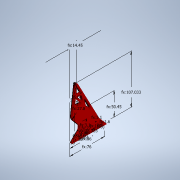
# Autodesk Inventor part: WeaponMountBasePlateV1
Saved by Autodesk Inventor 2020 (Build 240168000, 168)
## iProperties
Created: 2024-02-06
Part Number: WeaponMountBasePlateV1
Material: PETG
Document SubType Name: Modeling
Designer: smz3rm
Density: 1 g/cm^3
Appearance: Generic
Mass: 9.49681 g
Surface Area: 76.5782 cm^2
Volume: 9.49681 cm^3
WeaponHeight: 50.450 mm
SlotWidth: 6.000 mm
WeaponBite: 30.000 mm
WeaponMotorDia: 27.800 mm
SlotSpacing: 16.333 mm
SlotOffset: 2.000 mm
SlotHeight: 4.000 mm
SlotTolerance: 0.800 mm
WeaponMountBaseThinThickness: 1.000 mm
Height: 30.000 mm
BaseThickness: 3.000 mm
SideThickness: 6.000 mm
TopThickness: 1.000 mm
M3ScrewInsertBrim: 8.000 mm
M3ScrewDia: 3.100 mm
M3ScrewInsertDia: 4.000 mm
VM3ScrewInsertDia: 3.750 mm
FrontAngle: 45.00 deg
WeaponOpeningWidth: 15.000 mm
WeaponAssemblyWidth: 35.000 mm
WeaponCenterToMotorBack: 32.000 mm
WeaponMountThickness: 5.000 mm
WeaponDia: 88.900 mm
WeaponThickness: 3.000 mm
WeaponClearance: 10.000 mm
WeaponMotorShaftDia: 4.500 mm
WeaponMountWidth: 55.000 mm
Author: smz3rm
Autodesk Inventor part; units mm, degrees
ref_plane "YZ Plane" through (0, 0, 0) normal (1, 0, 0) x (0, 1, 0)
ref_plane "XZ Plane" through (0, 0, 0) normal (0, 1, 0) x (-1, 0, 0)
ref_plane "XY Plane" through (0, 0, 0) normal (0, 0, 1) x (1, 0, 0)
sketch "Sketch1" plane through (0, 0, 0) normal (1, 0, 0) x (0, 1, 0)
  line L0 (0, 0) -> (27, -27)
  line L1 (27, -27) -> (0, -27)
  line L2 (0, -27) -> (0, 0)
  line L3 (0, -76) -> (0, -27)
  arc A0 (52.1657, -0.6563) -> (59.496, -25.0037) centre (50.45, -14.45) ccw
  line L4 (6.4, -27) -> (1.6, -27)
  line L5 (1.6, -27) -> (1.6, -33.8)
  line L6 (1.6, -33.8) -> (6.4, -33.8)
  line L7 (6.4, -33.8) -> (6.4, -27)
  line L8 (1.6, -50.1333) -> (6.4, -50.1333)
  line L9 (6.4, -43.3333) -> (1.6, -43.3333)
  line L10 (1.6, -43.3333) -> (1.6, -50.1333)
  line L11 (6.4, -50.1333) -> (6.4, -43.3333)
  line L12 (1.6, -66.4667) -> (6.4, -66.4667)
  line L13 (6.4, -59.6667) -> (1.6, -59.6667)
  line L14 (1.6, -59.6667) -> (1.6, -66.4667)
  line L15 (6.4, -66.4667) -> (6.4, -59.6667)
  line L16 (0, -76) -> (59.496, -25.0037)
  arc A1 (108.2028, -12.2092) -> (107.3412, -7.5191) centre (107.0326, -10) ccw
  line L17 (52.1657, -0.6563) -> (107.3412, -7.5191)
  line L18 (19.7788, -59.0468) -> (108.2028, -12.2092)
  arc A2 (59.496, -25.0037) -> (52.1657, -0.6563) centre (50.45, -14.45) ccw
  arc A3 (61.4483, -27.2815) -> (64.6117, -5.2275) centre (50.45, -14.45) ccw
  line L19 (64.6117, -5.2275) -> (105.3972, -10.3004)
  line L20 (105.3972, -10.3004) -> (42.2134, -43.7685)
  line L21 (21.2075, -21.2075) -> (41.404, -3.8963)
  line L22 (27, -27) -> (21.2075, -21.2075)
  circle A4 centre (10, -30) radius 1.55
  circle A5 centre (10, -56) radius 1.55
  line L23 (61.4483, -27.2815) -> (42.2134, -43.7685)
  line L24 (59.496, -25.0037) -> (61.4483, -27.2815)
  point P0 (0, -25.1779)
  point P1 (1.6, -27)
  dimension "SlotWidth" = 6
  dimension "SlotSpacing" = 16.3333
  dimension "SlotTolerance" = 0.8
  dimension "d0" = 45
  dimension "d1" = 27
  dimension "d34" = 27.8
  dimension "d40" = 50.45
  dimension "d55" = 4.8
  dimension "d56" = 6.8
  dimension "d57" = 1.6
  dimension "d60" = 16.3333
  dimension "d65" = 5
  dimension "d66" = 10
  dimension "d67" = 107.0326
  dimension "d71" = 3
  dimension "d72" = 3
  dimension "d81" = 49
  dimension "d100" = 14.45
  dimension "d102" = 76
  dimension "d103" = 3.1
  dimension "d104" = 10
  dimension "d105" = 30
  dimension "d106" = 3.1
  dimension "d108" = 56
  dimension "d109" = 10
  dimension "d110" = 35
  constraints: 51 end point, 9 point on circle, 6 centre point, 6 tangent, 3 parallel, 3 perpendicular, 3 point on line, 2 horizontal, 2 vertical, 1 coincident, 1 collinear, 17 other
  measures "d0" angle of L2 L0
  measures "d1" distance of L0.end L1.end
  measures "d34" diameter of A0
  measures "d40" distance from line of L3 point (50.45, -14.45)
  measures "d55" distance of L6.end L5.end
  measures "d56" distance of L5.end L4.end
  measures "d57" distance between parallel lines of L3 L5
  measures "d60" distance of L5.end L8.start
  measures "d65" diameter of A1
  measures "d66" vertical distance of L0.start A1.centre
  measures "d67" distance from line of L3 A1.centre
  measures "d71" radial gap between concentric circles of A2 A3
  measures "d72" distance between parallel lines of L17 L19
  measures "d81" distance from line of L3.start L1
  measures "d100" vertical distance of point (50.45, -14.45) L0.start
  measures "d102" distance of L3.start L0.start
  measures "d103" diameter of A4
  measures "d104" distance from line of L2 A4.centre
  measures "d105" vertical distance of L0.start A4.centre
  measures "d106" diameter of A5
  measures "d108" vertical distance of L0.start A5.centre
  measures "d109" distance from line of L3 A5.centre
  measures "d110" angle of L17 L18
extrude "Extrusion1" add sketch "Sketch1" along normal blind 5 contours L0 L1 L2 | L21 A0 L16 L3 L1 L5 L6 L7 L0 | A0 A2 | L17 A1 L18 L16 A2
sketch "Sketch9" plane through (5, 0, 0) normal (1, 0, 0) x (0, 0, -1)
  line L0 (5.2275, 64.6117) -> (10.3004, 105.3972) projected
  line L1 (7.764, 85.0045) -> (27.2815, 61.4483)
  line L2 (27.2815, 61.4483) -> (21.1023, 85.0045)
  line L3 (10.3004, 105.3972) -> (43.7685, 42.2134) projected
  line L4 (7.764, 85.0045) -> (21.1023, 85.0045)
  line L5 (24.1099, 67.6272) -> (10.9548, 83.5045)
  line L6 (10.9548, 83.5045) -> (19.9451, 83.5045)
  line L7 (19.9451, 83.5045) -> (24.1099, 67.6272)
  line L8 (7.5097, 82.9603) -> (21.8624, 65.6377)
  line L9 (7.9505, 86.5045) -> (20.3078, 86.5045)
  line L10 (29.5161, 58.8413) -> (24.1745, 79.2046)
  line L11 (27.2815, 61.4483) -> (14.1292, 86.5045)
  arc A0 (27.2815, 61.4483) -> (5.2275, 64.6117) centre (14.45, 50.45) ccw projected
  line L12 (43.7685, 42.2134) -> (27.2815, 61.4483) projected
  point P0 (0, 0)
  point P1 (5.6914, 68.3412)
  point P2 (8.3929, 66.2272)
  dimension "d94" = 1.5
  dimension "d95" = 1.5
  dimension "d96" = 1.5
  dimension "d97" = 1.5
  constraints: 20 end point, 6 point on line, 3 parallel, 2 midpoint, 1 horizontal, 1 point on circle, 2 other
  measures "d94" distance between parallel lines of L1 L5
  measures "d95" distance between parallel lines of L1 L8
  measures "d96" distance between parallel lines of L9 L4
  measures "d97" distance between parallel lines of L10 L2
extrude "Extrusion9" add sketch "Sketch9" against normal up to surface (5 mm away) contours L0 L1 A0 L8 | L4 L11 L6 L5 L1 | L0 L9 L11 L4 | L11 L5 L7 L6 L4 L2 | L2 L3 L10 L12 | L11 L9 L3 L4
fillet "Fillet2" radius 10 2 edges at (2.5, 19.7788, -59.0468) (2.5, 21.2075, -21.2075)
sketch "Sketch7" plane through (5, 0, 0) normal (1, 0, 0) x (0, 0, -1)
  arc A0 (12.2092, 108.2028) -> (7.5191, 107.3412) centre (10, 107.0326) ccw projected
  line L0 (7.5191, 107.3412) -> (0.6563, 52.1657) projected
  arc A1 (0.6563, 52.1657) -> (3.8963, 41.404) centre (14.45, 50.45) ccw projected
  line L1 (3.8963, 41.404) -> (15.181, 28.2385) projected
  line L2 (76, 0) -> (59.7705, 18.9345) projected
  line L3 (58.5262, 20.7616) -> (12.2092, 108.2028) projected
  line L4 (66.4667, 1.6) -> (59.6667, 1.6) projected
  line L5 (27, 6.4) -> (33.8, 6.4) projected
  line L6 (27, 1.6) -> (27, 6.4) projected
  arc A2 (58.5262, 20.7616) -> (59.7705, 18.9345) centre (67.3631, 25.4424) ccw projected
  arc A3 (14.6595, 14.6595) -> (15.181, 28.2385) centre (7.5884, 21.7306) ccw projected
  line L7 (33.8, 6.4) -> (33.8, 1.6) projected
  line L8 (33.8, 1.6) -> (27, 1.6) projected
  line L9 (66.4667, 6.4) -> (66.4667, 1.6) projected
  line L10 (59.6667, 1.6) -> (59.6667, 6.4) projected
  line L11 (59.6667, 6.4) -> (66.4667, 6.4) projected
  line L12 (14.6595, 14.6595) -> (0, 0) projected
  line L13 (0, 0) -> (76, 0) projected
  point P0 (23.7912, 23.7912)
  point P1 (17.4514, 17.4514)
fillet "Fillet3" radius 0.5 24 edges at (5, 6.4, -30.4) (5, 4, -27) (5, 1.6, -30.4) (0, 4, -27) (0, 6.4, -30.4) (0, 1.6, -30.4) (5, 4, -33.8) (0, 4, -33.8) (5, 4, -43.3333) (0, 4, -43.3333) (5, 1.6, -46.7333) (5, 6.4, -46.7333) (0, 4, -50.1333) (5, 4, -50.1333) (5, 4, -59.6667) (5, 6.4, -63.0667) (5, 1.6, -63.0667) (5, 4, -66.4667) (0, 4, -66.4667) (0, 4, -59.6667) (0, 1.6, -63.0667) (0, 6.4, -63.0667) (0, 1.6, -46.7333) (0, 6.4, -46.7333)
sketch "Sketch8" plane through (5, 0, 0) normal (1, 0, 0) x (0, 0, -1)
  circle A0 centre (20, 12) radius 1.8
  point P0 (0, 0)
  dimension "d76" = 3.6
  dimension "d77" = 12
  dimension "d78" = 20
  constraints: 1 centre point
  measures "d76" diameter of A0
  measures "d77" vertical distance of point (0, 0) A0.centre
  measures "d78" horizontal distance of A0.centre point (0, 0)
extrude "Extrusion8" cut sketch "Sketch8" against normal through all
fillet "Fillet4" radius 1 12 edges at (2.5, 86.5045, -7.9505) (2.5, 86.5045, -20.3078) (2.5, 82.9603, -7.5097) (2.5, 79.2046, -24.1745) (2.5, 83.5045, -10.9548) (2.5, 83.5045, -19.9451) (2.5, 67.6272, -24.1099) (2.5, 64.6117, -5.2275) (2.5, 65.6377, -21.8624) (2.5, 42.2134, -43.7685) (2.5, 105.3972, -10.3004) (2.5, 58.8413, -29.5161)
equation "\"SlotWidth\" = 6"
equation "\"SlotSpacing\" = 16.33333"
equation "\"SlotTolerance\" = 0.8"
equation "\"d0\" = FrontAngle"
equation "\"d1\" = Height - BaseThickness"
equation "\"d34\" = WeaponMotorDia"
equation "\"WeaponHeight\" = 50.45"
equation "\"WeaponBite\" = 30"
equation "\"WeaponMotorDia\" = 27.8"
equation "\"SlotOffset\" = 2"
equation "\"SlotHeight\" = 4"
equation "\"WeaponMountBaseThinThickness\" = 1"
equation "\"WeaponBodyOffset\" = 77.9"
equation "\"WeaponLengthOffset\" = 162.55"
equation "\"BumpLengthOffset\" = 167"
equation "\"BumpHeight\" = 107.03261"
equation "\"WeaponMountRearAngle\" = 50deg"
equation "\"FrontAngle\" = 45deg"
equation "\"Height\" = 30"
equation "\"BaseThickness\" = 3"
body "Solid1"
